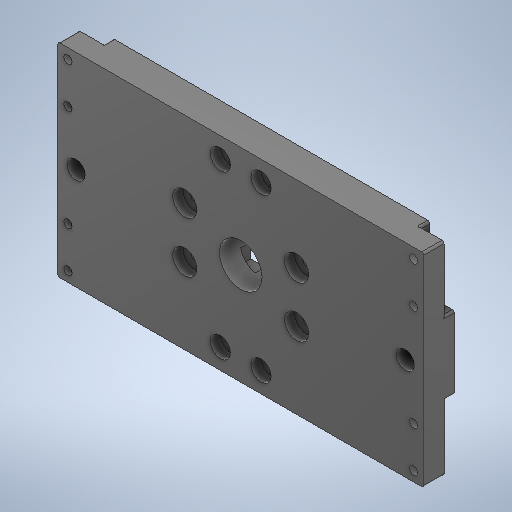
# Autodesk Inventor part: gripper_base
Saved by Autodesk Inventor 2026.2 (Build 302298010, 298A)
## iProperties
Created: 2026-04-12
Part Number: gripper_base
Material: ABS Plastic
Document SubType Name: Modeling
Designer: chris
Density: 1.06 g/cm^3
Appearance: Smooth - White
Author: chris
Autodesk Inventor part; units mm, degrees
ref_plane "YZ Plane" through (0, 0, 0) normal (1, 0, 0) x (0, 1, 0)
ref_plane "XZ Plane" through (0, 0, 0) normal (0, 1, 0) x (-1, 0, 0)
ref_plane "XY Plane" through (0, 0, 0) normal (0, 0, 1) x (1, 0, 0)
sketch "Sketch1" plane through (0, 0, 0) normal (0, 0, 1) x (1, 0, 0)
  line L0 (-90, -50) -> (90, -50)
  line L1 (90, -50) -> (90, 50)
  line L2 (90, 50) -> (-90, 50)
  line L3 (-90, 50) -> (-90, -50)
  line L4 (-90, -50) -> (90, 50) construction
  line L5 (90, -50) -> (-90, 50) construction
  point P0 (0, 0)
  dimension "d0" = 180
  dimension "d1" = 100
  constraints: 12 end point, 2 midpoint, 2 parallel, 1 horizontal, 1 perpendicular
  measures "d0" distance of L2.end L1.end
  measures "d1" distance of L1.end L0.end
extrude "Extrusion1" add sketch "Sketch1" along normal blind 10
sketch "Sketch2" plane through (0, 0, 10) normal (0, 0, 1) x (1, 0, 0)
  circle A0 centre (0, 0) radius 10.5
  dimension "d4" = 21
  constraints: 1 centre point, 1 coincident
  measures "d4" diameter of A0
extrude "Extrusion2" cut sketch "Sketch2" against normal through all
sketch "Sketch3" plane through (0, 0, 0) normal (0, 0, -1) x (-1, 0, 0)
  line L0 (-90, 18) -> (-78, 18)
  line L1 (-78, 18) -> (-78, 50)
  line L2 (-78, 50) -> (-90, 50)
  line L3 (-90, 50) -> (-90, 18)
  line L4 (78, 18) -> (90, 18)
  line L5 (90, 18) -> (90, 50)
  line L6 (90, 50) -> (78, 50)
  line L7 (78, 50) -> (78, 18)
  line L8 (78, -18) -> (90, -18)
  line L9 (90, -18) -> (90, -50)
  line L10 (90, -50) -> (78, -50)
  line L11 (78, -50) -> (78, -18)
  line L12 (-78, -18) -> (-90, -18)
  line L13 (-90, -18) -> (-90, -50)
  line L14 (-90, -50) -> (-78, -50)
  line L15 (-78, -50) -> (-78, -18)
  line L16 (-90, -50) -> (-90, 50) projected
  line L17 (-90, 50) -> (90, 50) projected
  line L18 (90, -50) -> (-90, -50) projected
  line L19 (90, 50) -> (90, -50) projected
  point P0 (0, 0)
  dimension "d7" = 32
  dimension "d8" = 12
  dimension "d9" = 12
  dimension "d10" = 32
  dimension "d11" = 12
  dimension "d12" = 32
  dimension "d13" = 12
  dimension "d14" = 32
  constraints: 32 end point, 8 collinear, 8 parallel, 4 horizontal, 4 perpendicular
  measures "d7" distance of L0.end L1.end
  measures "d8" distance of L0.start L0.end
  measures "d9" distance of L12.start L12.end
  measures "d10" distance of L14.end L12.start
  measures "d11" distance of L8.start L8.end
  measures "d12" distance of L10.end L8.start
  measures "d13" distance of L4.start L4.end
  measures "d14" distance of L6.end L4.start
extrude "Extrusion3" cut sketch "Sketch3" against normal blind 5 contours L3 L2 L1 L0 | L12 L15 L14 L13 | L6 L5 L4 L7 | L11 L8 L9 L10
sketch "Sketch4" plane through (0, 0, 10) normal (0, 0, 1) x (1, 0, 0)
  circle A0 centre (95, 45) radius 2.05 projected
  circle A1 centre (95, -45) radius 2.05 projected
  circle A2 centre (95, -25) radius 2.05 projected
  circle A3 centre (95, 25) radius 2.05 projected
  circle A4 centre (-95, 45) radius 2.05 projected
  circle A5 centre (-95, 25) radius 2.05 projected
  circle A6 centre (-95, -45) radius 2.05 projected
  circle A7 centre (-95, -25) radius 2.05 projected
  point P0 (0, 0)
hole "Hole1" at (95, 45, 10) at (95, 25, 10) at (95, -25, 10) at (95, -45, 10) at (-95, 45, 10) at (-95, 25, 10) at (-95, -25, 10) at (-95, -45, 10) direction (0, 0, -1) diameter 4.1 end through all
sketch "Sketch5" plane through (0, 0, 0) normal (0, 0, -1) x (-1, 0, 0)
  point P0 (0, 0)
sketch "Sketch6" plane through (0, 0, 0) normal (0, 0, -1) x (-1, 0, 0)
  line L0 (-10.1, -10.05) -> (10.1, -10.05)
  line L1 (10.1, -10.05) -> (10.1, 30.15)
  line L2 (10.1, 30.15) -> (-10.1, 30.15)
  line L3 (-10.1, 30.15) -> (-10.1, -10.05)
  line L4 (-10.1, -10.05) -> (10.1, 30.15) construction
  line L5 (10.1, -10.05) -> (-10.1, 30.15) construction
  point P0 (0, 0)
  point P1 (0, 10.05)
  dimension "d24" = 20.2
  dimension "d25" = 40.2
  dimension "d26" = 10.05
  constraints: 12 end point, 2 midpoint, 2 parallel, 1 horizontal, 1 perpendicular
  measures "d24" distance of L2.end L1.end
  measures "d25" distance of L0.end L1.end
  measures "d26" distance from line of L0 point (0, 0)
extrude "Extrusion4" cut sketch "Sketch6" against normal blind 5
sketch "Sketch7" plane through (0, 0, 10) normal (0, 0, 1) x (1, 0, 0)
  circle A0 centre (27.5, 12.5) radius 2.05 projected
  circle A1 centre (27.5, -12.5) radius 2.05 projected
  circle A2 centre (-27.5, 12.5) radius 2.05 projected
  circle A3 centre (-27.5, -12.5) radius 2.05 projected
  point P0 (0, 0)
hole "Hole2" at (-27.5, 12.5, 10) at (27.5, 12.5, 10) at (27.5, -12.5, 10) at (-27.5, -12.5, 10) direction (0, 0, -1) diameter 4.1 end through all
sketch "Sketch8" plane through (0, 0, 10) normal (0, 0, 1) x (1, 0, 0)
  circle A0 centre (-27.5, 12.5) radius 2.05 projected
  circle A1 centre (27.5, 12.5) radius 2.05 projected
  circle A2 centre (27.5, -12.5) radius 2.05 projected
  circle A3 centre (-27.5, -12.5) radius 2.05 projected
  circle A4 centre (-27.5, 12.5) radius 6
  circle A5 centre (27.5, 12.5) radius 6
  circle A6 centre (-27.5, -12.5) radius 6
  circle A7 centre (27.5, -12.5) radius 6
  point P0 (0, 0)
  dimension "d36" = 12
  dimension "d37" = 12
  dimension "d38" = 12
  dimension "d39" = 12
  constraints: 4 centre point, 4 coincident
  measures "d36" diameter of A4
  measures "d37" diameter of A5
  measures "d38" diameter of A6
  measures "d39" diameter of A7
extrude "Extrusion5" cut sketch "Sketch8" against normal blind 5 contours A0 | A1 | A3 | A4 | A5 | A6 | A7
sketch "Sketch9" plane through (0, 0, 10) normal (0, 0, 1) x (1, 0, 0)
  circle A0 centre (-85, 45) radius 2.05
  circle A1 centre (-85, 25) radius 2.05
  circle A2 centre (-85, -25) radius 2.05
  circle A3 centre (-85, -45) radius 2.05
  circle A4 centre (85, 45) radius 2.05
  circle A5 centre (85, 25) radius 2.05
  circle A6 centre (85, -25) radius 2.05
  circle A7 centre (85, -45) radius 2.05
  line L0 (90, 50) -> (-90, 50) projected
  line L1 (-90, -50) -> (90, -50) projected
  line L2 (-90, 50) -> (-90, -50) projected
  line L3 (90, -50) -> (90, 50) projected
  point P0 (0, 0)
  dimension "d42" = 4.1
  dimension "d43" = 4.1
  dimension "d44" = 4.1
  dimension "d45" = 4.1
  dimension "d46" = 4.1
  dimension "d47" = 4.1
  dimension "d48" = 4.1
  dimension "d49" = 4.1
  dimension "d50" = 5
  dimension "d51" = 25
  dimension "d52" = 25
  dimension "d53" = 5
  dimension "d54" = 5
  dimension "d55" = 25
  dimension "d56" = 25
  dimension "d57" = 5
  dimension "d58" = 5
  dimension "d59" = 5
  dimension "d60" = 5
  dimension "d61" = 5
  dimension "d62" = 5
  dimension "d63" = 5
  dimension "d64" = 5
  dimension "d65" = 5
  constraints: 8 centre point
  measures "d42" diameter of A0
  measures "d43" diameter of A1
  measures "d44" diameter of A2
  measures "d45" diameter of A3
  measures "d46" diameter of A4
  measures "d47" diameter of A5
  measures "d48" diameter of A6
  measures "d49" diameter of A7
  measures "d50" distance from line of L0 A0.centre
  measures "d51" distance from line of L0 A1.centre
  measures "d52" distance from line of L1 A2.centre
  measures "d53" distance from line of L1 A3.centre
  measures "d54" distance from line of L1 A7.centre
  measures "d55" distance from line of L1 A6.centre
  measures "d56" distance from line of L0 A5.centre
  measures "d57" distance from line of L0 A4.centre
  measures "d58" distance from line of L2 A0.centre
  measures "d59" distance from line of L2 A1.centre
  measures "d60" distance from line of L2 A2.centre
  measures "d61" distance from line of L2 A3.centre
  measures "d62" distance from line of L3 A4.centre
  measures "d63" distance from line of L3 A5.centre
  measures "d64" distance from line of L3 A6.centre
  measures "d65" distance from line of L3 A7.centre
extrude "Extrusion6" cut sketch "Sketch9" against normal through all contours A0 | A1 | A2 | A3 | A4 | A5 | A6 | A7
sketch "Sketch10" plane through (0, 0, 10) normal (0, 0, 1) x (1, 0, 0)
  circle A0 centre (81, 0) radius 4.5
  circle A1 centre (-81, 0) radius 4.5
  line L0 (90, -50) -> (90, 50) projected
  line L1 (-90, 50) -> (-90, -50) projected
  point P0 (0, 0)
  dimension "d68" = 9
  dimension "d69" = 9
  dimension "d70" = 9
  dimension "d71" = 9
  constraints: 2 centre point
  measures "d68" diameter of A0
  measures "d69" diameter of A1
  measures "d70" distance from line of L0 A0.centre
  measures "d71" distance from line of L1 A1.centre
extrude "Extrusion7" cut sketch "Sketch10" against normal blind 10
sketch "Sketch11" plane through (0, 0, 10) normal (0, 0, 1) x (1, 0, 0)
  circle A0 centre (-10, 40) radius 2.05
  circle A1 centre (10, 40) radius 2.05
  circle A2 centre (-10, -40) radius 2.05
  circle A3 centre (10, -40) radius 2.05
  line L0 (90, 50) -> (-90, 50) projected
  line L1 (-90, -50) -> (90, -50) projected
  point P0 (0, 0)
  dimension "d74" = 4.1
  dimension "d75" = 4.1
  dimension "d76" = 4.1
  dimension "d77" = 4.1
  dimension "d78" = 10
  dimension "d79" = 10
  dimension "d80" = 10
  dimension "d81" = 10
  dimension "d82" = 10
  dimension "d83" = 10
  dimension "d84" = 10
  dimension "d85" = 10
  constraints: 4 centre point
  measures "d74" diameter of A0
  measures "d75" diameter of A1
  measures "d76" diameter of A2
  measures "d77" diameter of A3
  measures "d78" distance from line of L0 A0.centre
  measures "d79" distance from line of L0 A1.centre
  measures "d80" distance from line of L1 A2.centre
  measures "d81" distance from line of L1 A3.centre
  measures "d82" horizontal distance of A2.centre point (0, 0)
  measures "d83" horizontal distance of point (0, 0) A3.centre
  measures "d84" horizontal distance of point (0, 0) A0.centre
  measures "d85" horizontal distance of point (0, 0) A1.centre
extrude "Extrusion8" cut sketch "Sketch11" against normal blind 10
sketch "Sketch12" plane through (0, 0, 10) normal (0, 0, 1) x (1, 0, 0)
  circle A0 centre (-10, 40) radius 2.05 projected
  circle A1 centre (10, 40) radius 2.05 projected
  circle A2 centre (-10, -40) radius 2.05 projected
  circle A3 centre (10, -40) radius 2.05 projected
  circle A4 centre (10, 40) radius 5
  circle A5 centre (-10, 40) radius 5
  circle A6 centre (10, -40) radius 5
  circle A7 centre (-10, -40) radius 5
  point P0 (0, 0)
  dimension "d88" = 10
  dimension "d89" = 10
  dimension "d90" = 10
  dimension "d91" = 10
  constraints: 4 centre point, 4 coincident
  measures "d88" diameter of A4
  measures "d89" diameter of A5
  measures "d90" diameter of A6
  measures "d91" diameter of A7
extrude "Extrusion9" cut sketch "Sketch12" against normal blind 5 contours A0 | A1 | A2 | A3 | A4 | A5 | A6 | A7
sketch "Sketch13" plane through (0, 0, 10) normal (0, 0, 1) x (1, 0, 0)
  circle A0 centre (10, -40) radius 5 projected
  circle A1 centre (10, 40) radius 5 projected
  circle A2 centre (-10, -40) radius 5 projected
  circle A3 centre (-10, 40) radius 5 projected
  circle A4 centre (81, 0) radius 4.5 projected
  circle A5 centre (-81, 0) radius 4.5 projected
  circle A6 centre (-85, -25) radius 2.05 projected
  circle A7 centre (85, -25) radius 2.05 projected
  circle A8 centre (85, 25) radius 2.05 projected
  circle A9 centre (-85, 25) radius 2.05 projected
  circle A10 centre (-85, -45) radius 2.05 projected
  circle A11 centre (85, -45) radius 2.05 projected
  circle A12 centre (85, 45) radius 2.05 projected
  circle A13 centre (-85, 45) radius 2.05 projected
  circle A14 centre (27.5, -12.5) radius 6 projected
  circle A15 centre (27.5, 12.5) radius 6 projected
  circle A16 centre (-27.5, -12.5) radius 6 projected
  circle A17 centre (-27.5, 12.5) radius 6 projected
  circle A18 centre (0, 0) radius 10.5 projected
  line L0 (90, -50) -> (90, 50) projected
  line L1 (90, 50) -> (-90, 50) projected
  line L2 (-90, 50) -> (-90, -50) projected
  line L3 (-90, -50) -> (90, -50) projected
extrude "Extrusion10" add sketch "Sketch13" along normal blind 5
sketch "Sketch14" plane through (-10, 40, 5) normal (0, 0, 1) x (1, 0, 0)
  circle A0 centre (0, 0) radius 2.05 projected
  circle A1 centre (0, 0) radius 5 projected
  circle A2 centre (20, 0) radius 2.05 projected
  circle A3 centre (20, 0) radius 5 projected
  circle A4 centre (-17.5, -27.5) radius 2.05 projected
  circle A5 centre (-17.5, -27.5) radius 6 projected
  circle A6 centre (37.5, -27.5) radius 2.05 projected
  circle A7 centre (37.5, -27.5) radius 6 projected
  circle A8 centre (-17.5, -52.5) radius 2.05 projected
  circle A9 centre (-17.5, -52.5) radius 6 projected
  circle A10 centre (37.5, -52.5) radius 6 projected
  circle A11 centre (37.5, -52.5) radius 2.05 projected
  circle A12 centre (0, -80) radius 2.05 projected
  circle A13 centre (0, -80) radius 5 projected
  circle A14 centre (20, -80) radius 2.05 projected
  circle A15 centre (20, -80) radius 5 projected
  point P0 (10, -40)
extrude "Extrusion11" add sketch "Sketch14" along normal blind 5
fillet "Fillet1" radius 1 12 edges at (90, 50, 10) (90, -50, 10) (-90, -50, 10) (-90, 50, 10) (90, -18, 2.5) (90, 18, 2.5) (78, -50, 2.5) (78, 50, 2.5) (-90, 18, 2.5) (-90, -18, 2.5) (-78, -50, 2.5) (-78, 50, 2.5)
body "Solid1"
